Lidar_support_v3 (Autodesk Fusion 360 design; units mm, degrees)
Autodesk Fusion 360 part; units mm, degrees
sketch "Esquisse1" plane through (0, 0, 0) normal (0, 0, 1) x (1, 0, 0) in component "Lidar"
  line L0 (12, 11.8) -> (-12, 11.8)
  line L1 (-12.8, 11) -> (-12.8, -11)
  line L2 (-12, -11.8) -> (12, -11.8)
  line L3 (12.8, -11) -> (12.8, 11)
  line L4 (12.8, 11.8) -> (-12.8, -11.8) construction
  line L5 (-12.8, 11.8) -> (12.8, -11.8) construction
  arc A0 (-12, 11.8) -> (-12.8, 11) centre (-12, 11) ccw
  arc A1 (12.8, 11) -> (12, 11.8) centre (12, 11) ccw
  arc A2 (12, -11.8) -> (12.8, -11) centre (12, -11) ccw
  arc A3 (-12.8, -11) -> (-12, -11.8) centre (-12, -11) ccw
  circle A4 centre (11, 10) radius 0.95
  line L6 (0, 0) -> (12.8, 0) construction
  line L7 (0, 0) -> (0, 11.8) construction
  circle A5 centre (11, -10) radius 0.95
  circle A6 centre (-11, 10) radius 0.95
  dimension "d1" = 25.6
  dimension "d2" = 23.6
  dimension "d3" = 0.8
  dimension "d4" = 1.9
  dimension "d5" = 1.8
  dimension "d6" = 1.8
  constraint horizontal L0
  constraint perpendicular L0 L1
  constraint parallel L0 L2
  constraint parallel L1 L3
  constraint coincident L4 L6.start
  constraint coincident L5 L6.start
  constraint coincident L6.start L7.start
  constraint coincident L5.start L1
  constraint coincident L5.start L0
  constraint tangent L1 A0
  constraint tangent L0 A0
  constraint coincident L4.start L3
  constraint coincident L4.start L0
  constraint tangent L3 A1
  constraint tangent L0 A1
  constraint equal A0 A1
  constraint coincident L5.end L2
  constraint coincident L5.end L3
  constraint tangent L2 A2
  constraint tangent L3 A2
  constraint equal A0 A2
  constraint coincident L4.end L2
  constraint coincident L4.end L1
  constraint tangent L2 A3
  constraint tangent L1 A3
  constraint equal A0 A3
  constraint midpoint L3 L6.end
  constraint midpoint L0 L7.end
  constraint symmetric A4 L6 A5
  constraint symmetric A4 L7 A6
  measures "d1" distance of L4.end L5.end
  measures "d2" distance of L5.start L4.end
  measures "d3" radius of A0
  measures "d4" diameter of A4
  measures "d5" distance of L0 A4.centre
  measures "d6" distance of L3 A4.centre
extrude "Extrusion1" add sketch "Esquisse1" along normal blind 1.6 makes body 1 in component "Lidar"
sketch "Esquisse2" plane through (0, 0, 1.6) normal (0, 0, 1) x (-1, 0, 0) in component "Lidar"
  circle A0 centre (-11, -10) radius 0.95
  circle A1 centre (11, -10) radius 0.95
  circle A2 centre (-11, 10) radius 0.95
  arc A3 (12.8, 11) -> (12, 11.8) centre (12, 11) ccw
  line L0 (12, 11.8) -> (-12, 11.8)
  arc A4 (-12, 11.8) -> (-12.8, 11) centre (-12, 11) ccw
  line L1 (-12.8, 11) -> (-12.8, -11)
  arc A5 (-12.8, -11) -> (-12, -11.8) centre (-12, -11) ccw
  line L2 (-12, -11.8) -> (12, -11.8)
  arc A6 (12, -11.8) -> (12.8, -11) centre (12, -11) ccw
  line L3 (12.8, -11) -> (12.8, 11)
  line L4 (9.07, 10.7) -> (-9.07, 10.7)
  line L5 (-9.07, 10.7) -> (-9.07, -10.7)
  line L6 (-9.07, -10.7) -> (9.07, -10.7)
  line L7 (9.07, -10.7) -> (9.07, 10.7)
  line L8 (9.07, 10.7) -> (-9.07, -10.7) construction
  line L9 (-9.07, 10.7) -> (9.07, -10.7) construction
  dimension "d9" = 18.14
  dimension "d10" = 21.4
  constraint horizontal L4
  constraint perpendicular L4 L5
  constraint parallel L4 L6
  constraint parallel L5 L7
  constraint coincident L8 origin
  constraint coincident L9 origin
  measures "d9" distance of L5.end L6.end
  measures "d10" distance of L4.end L5.end
extrude "Extrusion2" add sketch "Esquisse2" along normal blind 5.5 contours L4 L5 L6 L7 bodies 1 in component "Lidar"
sketch "Esquisse1 (2)" plane through (0, 0, 1.6) normal (0, 0, 1) x (-1, 0, 0) in component "Support"
  line L0 (9.07, -10.7) -> (-9.07, -10.7)
  line L1 (-9.07, -10.7) -> (-9.07, 10.7)
  line L2 (-9.07, 10.7) -> (9.07, 10.7)
  line L3 (9.07, 10.7) -> (9.07, -10.7)
  arc A0 (12.8, 11) -> (12, 11.8) centre (12, 11) ccw
  line L4 (12, 11.8) -> (-12, 11.8)
  arc A1 (-12, 11.8) -> (-12.8, 11) centre (-12, 11) ccw
  line L5 (-12.8, 11) -> (-12.8, -11)
  arc A2 (-12.8, -11) -> (-12, -11.8) centre (-12, -11) ccw
  line L6 (-12, -11.8) -> (12, -11.8)
  arc A3 (12, -11.8) -> (12.8, -11) centre (12, -11) ccw
  line L7 (12.8, -11) -> (12.8, 11)
  line L8 (-9.17, -10.8) -> (9.17, -10.8)
  line L9 (9.17, -10.8) -> (9.17, 10.8)
  line L10 (9.17, 10.8) -> (-9.17, 10.8)
  line L11 (-9.17, 10.8) -> (-9.17, -10.8)
  line L12 (-9.17, -10.8) -> (9.17, 10.8) construction
  line L13 (9.17, -10.8) -> (-9.17, 10.8) construction
  line L14 (-17.9, -16.9) -> (17.9, -16.9)
  line L15 (17.9, -16.9) -> (17.9, 16.9)
  line L16 (17.9, 16.9) -> (-17.9, 16.9)
  line L17 (-17.9, 16.9) -> (-17.9, -16.9)
  line L18 (-17.9, -16.9) -> (17.9, 16.9) construction
  line L19 (17.9, -16.9) -> (-17.9, 16.9) construction
  line L20 (-12.9, -11.9) -> (12.9, -11.9)
  line L21 (12.9, -11.9) -> (12.9, 11.9)
  line L22 (12.9, 11.9) -> (-12.9, 11.9)
  line L23 (-12.9, 11.9) -> (-12.9, -11.9)
  line L24 (-12.9, -11.9) -> (12.9, 11.9) construction
  line L25 (12.9, -11.9) -> (-12.9, 11.9) construction
  line L26 (0, 0) -> (0, -16.9) construction
  line L27 (0, 0) -> (-17.9, 0) construction
  dimension "d13" = 0.1
  dimension "d14" = 0.1
  dimension "d17" = 0.1
  dimension "d18" = 0.1
  dimension "d19" = 5
  dimension "d20" = 5
  constraint horizontal L8
  constraint perpendicular L8 L9
  constraint parallel L8 L10
  constraint parallel L9 L11
  constraint coincident L12 L26.start
  constraint coincident L13 L26.start
  constraint coincident L26.start L27.start
  constraint horizontal L14
  constraint perpendicular L14 L15
  constraint parallel L14 L16
  constraint parallel L15 L17
  constraint coincident L18 L26.start
  constraint coincident L19 L26.start
  constraint horizontal L20
  constraint perpendicular L20 L21
  constraint parallel L20 L22
  constraint parallel L21 L23
  constraint coincident L24 L26.start
  constraint coincident L25 L26.start
  constraint midpoint L14 L26.end
  constraint midpoint L17 L27.end
  measures "d13" distance of L1 L11
  measures "d14" distance of L0 L8
  measures "d17" distance of L6 L20
  measures "d18" distance of L5 L23
  measures "d19" distance of L14 L20
  measures "d20" distance of L17 L23
extrude "Extrusion1'" add sketch "Esquisse1 (2)" along normal blind 1 separate body contours A0 L4 A1 L5 A2 L6 A3 L7 | L14 L15 L16 L17 | L20 L21 L22 L23 makes body 2 in component "Support"
extrude "Extrusion3" add sketch "Esquisse1 (2)" against normal blind 10 contours L14 L15 L16 L17 bodies 2 in component "Support"
sketch "Esquisse3" plane through (12.9, 0, 0) normal (-1, 0, 0) x (0, -1, 0)
  line L0 (11.9, 1.6) -> (-11.9, 1.6)
  line L1 (-11.9, 1.6) -> (-11.9, -8.4)
  line L2 (-11.9, -8.4) -> (11.9, -8.4)
  line L3 (11.9, -8.4) -> (11.9, 1.6)
  line L4 (-11.9, 1.6) -> (11.9, -5.6764)
  line L5 (-11.9, 1.6) -> (5.6356, 1.6) construction
  line L6 (11.9, -5.6764) -> (11.9, 1.6)
  line L7 (11.9, 1.6) -> (-11.9, 1.6)
  dimension "d40" = 17
  constraint horizontal L5
  constraint coincident L0.end L1.start
  constraint coincident L0.start L3.end
  constraint perpendicular L6 L7
  measures "d40" angle of L4 L5
extrude "Extrusion7" add sketch "Esquisse3" along normal blind 25.8 contours L0 L3 L4 L6 L7 bodies 2 in component "Support"
extrude "Extrusion8" cut sketch "Esquisse1 (2)" against normal through all contours L0 L1 L2 L3 bodies 2 in component "Support"
sketch "Esquisse6" plane through (0, 0, -8.4) normal (0, 0, -1) x (1, 0, 0) in component "Support"
  line L0 (12.9, 11.9) -> (12.9, -11.9)
  line L1 (12.9, -11.9) -> (-12.9, -11.9)
  line L2 (-12.9, -11.9) -> (-12.9, 11.9)
  line L3 (-12.9, 11.9) -> (12.9, 11.9)
  line L4 (17.9, -16.9) -> (17.9, 16.9)
  line L5 (17.9, 16.9) -> (-17.9, 16.9)
  line L6 (-17.9, 16.9) -> (-17.9, -16.9)
  line L7 (-17.9, -16.9) -> (17.9, -16.9)
  circle A0 centre (-14.9, 13.9) radius 1.7
  line L8 (0, 0) -> (0, 7.5048) construction
  line L9 (0, 0) -> (7.5594, 0) construction
  circle A1 centre (14.9, 13.9) radius 1.7
  circle A2 centre (14.9, -13.9) radius 1.7
  circle A3 centre (-14.9, -13.9) radius 1.7
  dimension "d44" = 3.4
  dimension "d45" = 3
  dimension "d46" = 3
  constraint coincident L8.start L9.start
  constraint perpendicular L3 L8
  constraint perpendicular L8 L9
  constraint symmetric A0 L8 A1
  constraint symmetric A0 L9 A3
  constraint symmetric L9 A1 A2
  measures "d44" diameter of A0
  measures "d45" distance of L5 A0.centre
  measures "d46" distance of L6 A0.centre
extrude "Extrusion9" cut sketch "Esquisse6" against normal through all contours A0 | A1 | A2 | A3 bodies 2 in component "Support"
component "Lidar" placed x (1, 0, 0) y (0, 1, 0) z (0, 0, 1) at (0, 0, 0)
component "Support" placed x (1, 0, 0) y (0, 1, 0) z (0, 0, 1) at (0, 0, 0)
equation "d6 = d5"
equation "d46 = d45"
